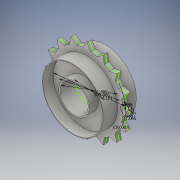
# Autodesk Inventor part: plastic drive gear
Saved by Autodesk Inventor 2016 (Build 200138000, 138)
## iProperties
Created: 2015-10-09
Part Number: plastic drive gear
Material: Generic
Document SubType Name: Modeling
Designer: Delta
Density: 1 g/cm^3
Appearance: Default
Author: Delta
Autodesk Inventor part; units mm, degrees
ref_plane "YZ Plane" through (0, 0, 0) normal (1, 0, 0) x (0, 1, 0)
ref_plane "XZ Plane" through (0, 0, 0) normal (0, 1, 0) x (-1, 0, 0)
ref_plane "XY Plane" through (0, 0, 0) normal (0, 0, 1) x (1, 0, 0)
sketch "Sketch1" plane through (0, 0, 0) normal (0, 0, 1) x (1, 0, 0)
  circle A0 centre (0, 0) radius 12.7
  circle A1 centre (0, 0) radius 12.446
  circle A2 centre (0, 0) radius 6.35
  circle A3 centre (0, 0) radius 5.8601
  circle A4 centre (0, 0) radius 15
  line L0 (15, 0) -> (17.5, 0)
  line L1 (15, 0) -> (17.5, 0) construction
  line L2 (17.5, 0) -> (15, 0)
  line L3 (17.5, 0) -> (14.9086, 1.6536)
  line L4 (17.5, 0) -> (14.9086, -1.6536)
  line L5 (14.9086, 1.6536) -> (14.9086, -1.6536)
  line L6 (13.1409, 7.233) -> (14.4065, 4.1775)
  line L7 (16.1679, 6.697) -> (13.1409, 7.233)
  line L8 (16.1679, 6.697) -> (14.4065, 4.1775)
  line L9 (9.3727, 11.7112) -> (11.7112, 9.3727)
  line L10 (12.3744, 12.3744) -> (9.3727, 11.7112)
  line L11 (12.3744, 12.3744) -> (11.7112, 9.3727)
  line L12 (4.1775, 14.4065) -> (7.233, 13.1409)
  line L13 (6.697, 16.1679) -> (4.1775, 14.4065)
  line L14 (6.697, 16.1679) -> (7.233, 13.1409)
  line L15 (-1.6536, 14.9086) -> (1.6536, 14.9086)
  line L16 (0, 17.5) -> (-1.6536, 14.9086)
  line L17 (0, 17.5) -> (1.6536, 14.9086)
  line L18 (-7.233, 13.1409) -> (-4.1775, 14.4065)
  line L19 (-6.697, 16.1679) -> (-7.233, 13.1409)
  line L20 (-6.697, 16.1679) -> (-4.1775, 14.4065)
  line L21 (-11.7112, 9.3727) -> (-9.3727, 11.7112)
  line L22 (-12.3744, 12.3744) -> (-11.7112, 9.3727)
  line L23 (-12.3744, 12.3744) -> (-9.3727, 11.7112)
  line L24 (-14.4065, 4.1775) -> (-13.1409, 7.233)
  line L25 (-16.1679, 6.697) -> (-14.4065, 4.1775)
  line L26 (-16.1679, 6.697) -> (-13.1409, 7.233)
  line L27 (-14.9086, -1.6536) -> (-14.9086, 1.6536)
  line L28 (-17.5, 0) -> (-14.9086, -1.6536)
  line L29 (-17.5, 0) -> (-14.9086, 1.6536)
  line L30 (-13.1409, -7.233) -> (-14.4065, -4.1775)
  line L31 (-16.1679, -6.697) -> (-13.1409, -7.233)
  line L32 (-16.1679, -6.697) -> (-14.4065, -4.1775)
  line L33 (-9.3727, -11.7112) -> (-11.7112, -9.3727)
  line L34 (-12.3744, -12.3744) -> (-9.3727, -11.7112)
  line L35 (-12.3744, -12.3744) -> (-11.7112, -9.3727)
  line L36 (-4.1775, -14.4065) -> (-7.233, -13.1409)
  line L37 (-6.697, -16.1679) -> (-4.1775, -14.4065)
  line L38 (-6.697, -16.1679) -> (-7.233, -13.1409)
  line L39 (1.6536, -14.9086) -> (-1.6536, -14.9086)
  line L40 (0, -17.5) -> (1.6536, -14.9086)
  line L41 (0, -17.5) -> (-1.6536, -14.9086)
  line L42 (7.233, -13.1409) -> (4.1775, -14.4065)
  line L43 (6.697, -16.1679) -> (7.233, -13.1409)
  line L44 (6.697, -16.1679) -> (4.1775, -14.4065)
  line L45 (11.7112, -9.3727) -> (9.3727, -11.7112)
  line L46 (12.3744, -12.3744) -> (11.7112, -9.3727)
  line L47 (12.3744, -12.3744) -> (9.3727, -11.7112)
  line L48 (14.4065, -4.1775) -> (13.1409, -7.233)
  line L49 (16.1679, -6.697) -> (14.4065, -4.1775)
  line L50 (16.1679, -6.697) -> (13.1409, -7.233)
  dimension "d1" = 25.4
  dimension "d2" = 24.892
  dimension "d3" = 12.7
  dimension "d22" = 30
  dimension "d24" = 2.5
  dimension "d25" = 0
  dimension "d26" = 3.0741
  dimension "d27" = 1.6536
  dimension "d30" = 360
  constraints: 102 end point, 5 centre point, 4 coincident, 4 point on circle, 2 horizontal, 1 collinear, 1 vertical, 97 other
  measures "d1" diameter of A0
  measures "d2" diameter of A1
  measures "d3" diameter of A2
  measures "d22" diameter of A4
  measures "d24" distance of L0.start L0.end
  measures "d25" distance between parallel lines of L0 L1
  measures "d26" distance of L1.end L3.end
  measures "d27" vertical distance of L1.end L4.end
extrude "Extrusion1" [suppressed]
extrude "Extrusion2" add sketch "Sketch1" along normal blind 6.858 and the other way blind 6.858 contours A0
extrude "Extrusion3" add sketch "Sketch1" along normal blind 2.54 and the other way blind 2.54 contours A1
extrude "Extrusion4" add sketch "Sketch1" along normal blind 6.35 and the other way blind 6.35 contours A2
fillet "Fillet1" [suppressed]
fillet "Fillet2" [suppressed]
extrude "Extrusion5" add sketch "Sketch1" along normal mid plane 2 contours L0 L4 A4 | A4 L3 L0 | L6 A4 | A4 L7 L8 | L49 L50 A4 | A4 L48 | L9 A4 | A4 L10 L11 | L46 L47 A4 | A4 L45 | L12 A4 | A4 L13 L14 | L43 L44 A4 | A4 L42 | L15 A4 | A4 L16 L17 | L40 L41 A4 | A4 L39 | L18 A4 | A4 L19 L20 | L37 L38 A4 | A4 L36 | L21 A4 | A4 L22 L23 | L34 L35 A4 | A4 L33 | L24 A4 | A4 L25 L26 | L31 L32 A4 | A4 L30 | L27 A4 | A4 L28 L29
extrude "Extrusion6" add sketch "Sketch1" along normal mid plane 2 contours L5 A4 L48 L45 L42 L39 L36 L33 L30 L27 L24 L21 L18 L15 L12 L9 L6 | L6 A4 | A4 L48 | L9 A4 | A4 L45 | L12 A4 | A4 L42 | L15 A4 | A4 L39 | L18 A4 | A4 L36 | L21 A4 | A4 L33 | L24 A4 | A4 L30 | L27 A4
body "Solid1"
